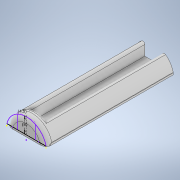
# Autodesk Inventor part: LED arm guard
Saved by Autodesk Inventor 2020 (Build 240168000, 168)
## iProperties
Created: 2021-05-17
Part Number: LED arm guard
Material: Generic
Document SubType Name: Modeling
Designer: Steven
Density: 1 g/cm^3
Appearance: Default
Author: Steven
Autodesk Inventor part; units mm, degrees
ref_plane "YZ Plane" through (0, 0, 0) normal (1, 0, 0) x (0, 1, 0)
ref_plane "XZ Plane" through (0, 0, 0) normal (0, 1, 0) x (-1, 0, 0)
ref_plane "XY Plane" through (0, 0, 0) normal (0, 0, 1) x (1, 0, 0)
sketch "Sketch1" plane through (0, 0, 0) normal (0, 1, 0) x (-1, 0, 0)
  line L0 (0, 0) -> (-20, 0)
  line L1 (-20, 0) -> (-20, -65)
  line L2 (-20, -65) -> (0, -65)
  line L3 (0, -65) -> (0, 0)
  dimension "d0" = 20
  dimension "d1" = 65
  constraints: 8 end point, 2 horizontal, 2 perpendicular
  measures "d0" distance of L0.start L0.end
  measures "d1" distance of L0.end L1.end
extrude "Extrusion1" add sketch "Sketch1" along normal blind 1
sketch "Sketch2" plane through (0, 0, 0) normal (0, 0, 1) x (1, 0, 0)
  line L0 (0, 1) -> (20, 1) construction
  line L1 (20, 0) -> (20, 1)
  line L2 (0, 1) -> (20, 1)
  line L3 (10, 1) -> (10, 9) construction
  arc A0 (20, 1) -> (0, 1) centre (10, -1.25) ccw
  line L4 (10, 9) -> (5.5, 9) construction
  line L5 (10, 9) -> (14.5, 9) construction
  line L6 (14.5, 9) -> (14.5, 7.95937) construction
  line L7 (5.5, 9) -> (5.5, 7.95937) construction
  line L8 (14.5, 7.95937) -> (14.5, 1)
  line L9 (5.5, 7.95937) -> (5.5, 1)
  point P0 (0, 0)
  point P1 (3, 1)
  point P2 (16.238791, 1)
  dimension "d12" = 8
  dimension "d13" = 4.5
  constraints: 16 end point, 5 point on circle, 4 point on line, 4 vertical, 2 perpendicular, 1 centre point, 1 horizontal, 1 midpoint, 1 symmetric about line, 1 tangent
  measures "d12" distance of L3.start L3.end
  measures "d13" distance of L3.end L4.end
extrude "Extrusion2" add sketch "Sketch2" against normal up to surface (65 mm away) contours A0 L9 L2 | L8 A0 L2
extrude "Extrusion3" add sketch "Sketch2" against normal blind 5
fillet "Fillet3" radius 3 1 edges at (10, 9, 0)
fillet "Fillet4" radius 1 5 edges at (14.5, 7.9594, -35) (20, 0.6638, -2.3625) (20, 1, -34) (5.5, 7.9594, -35) (10, 9, -5)
body "Solid1"
